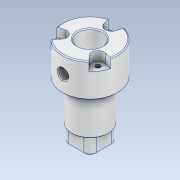
# Autodesk Inventor part: SteeringShaft
Saved by Autodesk Inventor 2020 (Build 240168000, 168)
## iProperties
Created: 2019-12-15
Part Number: SteeringShaft
Material: Aluminum 6061
Document SubType Name: Modeling
Designer: Kjell
Density: 2.7 g/cm^3
Appearance: Aluminum - Flat
Mass: 9.28499 g
Surface Area: 24.6296 cm^2
Volume: 3.43888 cm^3
Author: Kjell
Autodesk Inventor part; units mm, degrees
ref_plane "YZ Plane" through (0, 0, 0) normal (1, 0, 0) x (0, 1, 0)
ref_plane "XZ Plane" through (0, 0, 0) normal (0, 1, 0) x (-1, 0, 0)
ref_plane "XY Plane" through (0, 0, 0) normal (0, 0, 1) x (1, 0, 0)
sketch "Sketch2" plane through (0, 0, 0) normal (0, 0, 1) x (1, 0, 0)
  circle A0 centre (0, 0) radius 9
  dimension "d0" = 18
  constraints: 1 centre point, 1 coincident
  measures "d0" diameter of A0
extrude "Extrusion1" add sketch "Sketch2" against normal blind 11
sketch "Sketch3" plane through (0, 0, -11) normal (0, 0, -1) x (-1, 0, 0)
  circle A0 centre (0, 0) radius 9 projected
  circle A1 centre (0, 0) radius 5.975
  dimension "ShaftDia" = 11.95
  constraints: 1 centre point, 1 coincident
  measures "ShaftDia" diameter of A1
extrude "Extrusion2" add sketch "Sketch3" along normal blind 13 contours A1
sketch "Sketch4" plane through (0, 0, 0) normal (0, 0, 1) x (1, 0, 0)
  circle A0 centre (0, 0) radius 9 projected
  constraints: 1 coincident
hole "Hole1" at (0, 0, 0) direction (0, 0, -1) diameter 8.05 depth 15
sketch "Sketch5" plane through (0, 0, -24) normal (0, 0, -1) x (-1, 0, 0)
  circle A0 centre (0, 0) radius 5.975 projected
  line L0 (-2.5, 4.5) -> (2.5, 4.5)
  line L1 (4.5, 2.5) -> (4.5, -2.5)
  line L2 (2.5, -4.5) -> (-2.5, -4.5)
  line L3 (-4.5, -2.5) -> (-4.5, 2.5)
  line L4 (-4.5, 4.5) -> (4.5, -4.5) construction
  line L5 (4.5, 4.5) -> (-4.5, -4.5) construction
  arc A1 (4.5, 2.5) -> (2.5, 4.5) centre (2.5, 2.5) ccw
  arc A2 (2.5, -4.5) -> (4.5, -2.5) centre (2.5, -2.5) ccw
  arc A3 (-4.5, -2.5) -> (-2.5, -4.5) centre (-2.5, -2.5) ccw
  arc A4 (-2.5, 4.5) -> (-4.5, 2.5) centre (-2.5, 2.5) ccw
  dimension "d13" = 9
  dimension "d14" = 2
  constraints: 12 end point, 8 point on circle, 8 point on line, 8 tangent, 4 centre point, 3 equal radius, 2 midpoint, 2 parallel, 2 perpendicular, 1 horizontal
  measures "d13" distance of L4.start L5.start
  measures "d14" radius of A1
extrude "Extrusion3" add sketch "Sketch5" along normal blind 5 contours L0 A1 L1 A2 L2 A3 L3 A4
sketch "Sketch6" plane through (0, 0, -29) normal (0, 0, -1) x (-1, 0, 0)
  circle A0 centre (0, 0) radius 5.975 projected
  constraints: 1 coincident
hole "Hole2" at (0, 0, -29) direction (0, 0, 1) diameter 4.917 depth 12 tip angle 118 thread size "M6x1" class "6H" standard "ISO Metric profile"
ref_plane "Work Plane1" through (0, -9, 0) normal (0, -1, 0) x (1, 0, 0)
sketch "Sketch7" plane through (0, -9, 0) normal (0, -1, 0) x (1, 0, 0)
  line L0 (-9, -11) -> (9, -11) projected
  line L1 (9, 0) -> (-9, 0) projected
  point P0 (0, 0)
  point P1 (0, -5.5)
  dimension "d36" = 5.5
  constraints: 1 vertical alignment
  measures "d36" distance from line of point (0, -5.5) L0
hole "Hole3" at (0, -9, -5.5) direction (0, 1, 0) diameter 3.242 end up to face face through (0, 0, -7.5) facing (0, 0, 1) round with radius 4.025 far side no thread size "M4x0.7" class "6H" standard "ISO Metric profile"
chamfer "Chamfer1" distance 0.3 angle 45 15 edges at (-9, 0, 0) (0, 4.025, 0) (1.621, -8.8528, -5.5) (-1.621, -8.8528, -5.5) (-9, 0, -11) (5.975, 0, -24) (4.5, 0, -29) (3.9142, -3.9142, -29) (0, -4.5, -29) (-3.9142, -3.9142, -29) (-4.5, 0, -29) (-3.9142, 3.9142, -29) (0, 4.5, -29) (3.9142, 3.9142, -29) (0, -2.4585, -29)
sketch "Sketch8" plane through (0, 0, 0) normal (0, 0, 1) x (1, 0, 0)
  circle A0 centre (0, 0) radius 8.7 projected
  circle A1 centre (0, 0) radius 4.325 projected
  circle A2 centre (0, 0) radius 7 construction
  line L0 (0, 0) -> (0, 14.9328) construction
  circle A3 centre (0, 0) radius 9 projected
  line L1 (-1.9166, 6.4286) -> (-2.5714, 8.6248)
  line L2 (1.9166, 6.4286) -> (2.5714, 8.6248)
  arc A4 (-1.9795, 6.7143) -> (1.9795, 6.7143) centre (0, 7) ccw
  line L3 (-4.609, -4.8741) -> (-6.1836, -6.5393)
  arc A5 (-4.825, -5.0714) -> (-6.8045, -1.6429) centre (-6.0622, -3.5) ccw
  line L4 (-6.5256, -1.5544) -> (-8.755, -2.0855)
  line L5 (6.5256, -1.5544) -> (8.755, -2.0855)
  arc A6 (6.8045, -1.6429) -> (4.825, -5.0714) centre (6.0622, -3.5) ccw
  line L6 (4.609, -4.8741) -> (6.1836, -6.5393)
  point P0 (5.9775, -6.3214)
  point P1 (8.4632, -2.016)
  point P2 (2.4857, 8.3373)
  point P3 (-2.4857, 8.3373)
  point P4 (-8.4632, -2.016)
  point P5 (-5.9775, -6.3214)
  dimension "d37" = 14
  dimension "d41" = 360
  constraints: 17 point on circle, 14 end point, 4 centre point, 2 line through centre, 2 tangent, 1 coincident, 1 point on line, 1 vertical, 31 other
  measures "d37" diameter of A2
extrude "Extrusion4" cut sketch "Sketch8" against normal blind 3 contours L2 A4 L1 A0 | A0 L1 A3 L2 | L5 A3 L6 A0 | A0 L6 A6 L5 | L4 A5 L3 A0 | A0 L3 A3 L4
sketch "Sketch9" plane through (0, 0, -3) normal (0, 0, 1) x (1, 0, 0)
  arc A0 (6.5256, -1.5544) -> (4.609, -4.8741) centre (6.0622, -3.5) ccw projected
  arc A1 (-1.9166, 6.4286) -> (1.9166, 6.4286) centre (0, 7) ccw projected
  arc A2 (-4.609, -4.8741) -> (-6.5256, -1.5544) centre (-6.0622, -3.5) ccw projected
  point P0 (0, 0)
  constraints: 3 coincident
hole "Hole4" at (6.0622, -3.5, -3) at (0, 7, -3) at (-6.0622, -3.5, -3) direction (0, 0, -1) diameter 1.567 depth 5 tip angle 118 thread size "M2x0.4" class "6H" standard "ISO Metric profile"
body "Solid1"
